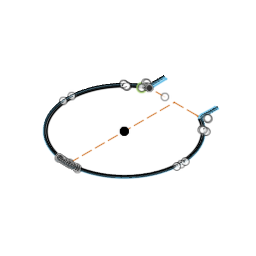
E-Baike Kunstoff abdeckung Schloss v12 (Autodesk Fusion 360 design; units mm, degrees)
Autodesk Fusion 360 part; units mm, degrees
note: some values were not read from the file. Set by a fixed rule: which sketch regions a step uses.
sketch "Skizze3" plane through (0, 0, 0) normal (0, 0, 1) x (1, 0, 0)
  line L0 (52.5263, 0.0019) -> (52.3815, 0.0019) construction
  line L1 (52.3815, 0.0019) -> (52.3815, -3.9178)
  line L2 (52.3815, 0.0019) -> (52.3815, 3.8983)
  arc A0 (37.2241, 37.4698) -> (37.51, 36.7698) centre (38.2241, 37.4698) ccw
  arc A1 (34.4473, 37.4285) -> (34.7597, 36.7024) centre (35.4473, 37.4285) ccw
  line L3 (-52.3815, 0.0019) -> (-52.3815, -3.9178)
  line L4 (-52.3815, 0.0019) -> (-52.3815, 3.8983)
  arc A2 (-34.7597, 36.7024) -> (-34.4473, 37.4285) centre (-35.4473, 37.4285) ccw
  arc A3 (-37.51, 36.7698) -> (-37.2241, 37.4698) centre (-38.2241, 37.4698) ccw
  line L5 (0, -50.55) -> (0, 46.165) construction
  line L6 (-25.0003, 48.4886) -> (-24.9973, 61.165)
  line L7 (25.0009, 48.4892) -> (25.0009, 61.165)
  line L8 (-24.9973, 61.165) -> (-24.3973, 61.1649)
  line L9 (25.0009, 61.165) -> (24.4009, 61.165)
  line L10 (23.8294, 48.6654) -> (24.4009, 61.165)
  line L11 (-23.8287, 48.6648) -> (-24.3973, 61.1649)
  line L12 (24.4009, 61.165) -> (22.5009, 61.165)
  line L13 (-24.3973, 61.1649) -> (-22.4973, 61.1644)
  arc A4 (-26.748, 42.8934) -> (-26.748, 42.8934) centre (0, 0) ccw
  arc A5 (-25.8336, 45.0137) -> (25.8341, 45.0134) centre (0, 0) ccw
  line L14 (-8.6883, 46.1611) -> (-20.5959, 46.164) construction
  line L15 (0, 46.165) -> (20.5936, 46.165) construction
  arc A6 (-25.8336, 45.0137) -> (-23.8287, 48.6648) centre (-27.8246, 48.483) ccw
  arc A7 (-26.9472, 45.0566) -> (-25.0003, 48.4886) centre (-29.0003, 48.4895) ccw
  arc A8 (25.0009, 48.4892) -> (26.9477, 45.0563) centre (29.0009, 48.4892) ccw
  arc A9 (23.8294, 48.6654) -> (25.8341, 45.0134) centre (27.8252, 48.4827) ccw
  line L16 (20.5936, 46.165) -> (22.0936, 46.165) construction
  line L17 (-20.5959, 46.164) -> (-22.0959, 46.164) construction
  line L18 (22.0936, 46.165) -> (22.0936, 45.4662) construction
  line L19 (-22.0959, 46.164) -> (-22.0959, 45.4651) construction
  line L20 (22.1899, 49.1795) -> (22.5009, 61.165)
  line L21 (-22.1908, 49.1767) -> (-22.4973, 61.1644)
  arc A10 (-25.198, 43.822) -> (25.1971, 43.8224) centre (0, 0) ccw
  arc A11 (52.3815, 3.5258) -> (26.9477, 45.0563) centre (0, 0) ccw
  arc A12 (-26.9472, 45.0566) -> (-52.3815, 3.5258) centre (0, 0) ccw
  arc A13 (-52.3815, -3.5258) -> (52.3815, -3.5258) centre (0, 0) ccw
  arc A14 (-25.198, 43.822) -> (-22.1908, 49.1767) centre (-28.1889, 49.0234) ccw
  arc A15 (22.1899, 49.1795) -> (25.1971, 43.8224) centre (28.1879, 49.0239) ccw
  line L22 (8.6033, -51.817) -> (8.6033, -51.7903) construction
  line L23 (-8.6033, -51.817) -> (-8.6033, -51.7903) construction
  point P0 (-25.0009, 46.165)
  point P1 (-25.0009, 46.165)
  point P2 (-25.7438, 46.1667)
  point P3 (-22.9574, 46.0854)
  dimension "d26" = 1
  dimension "d34" = 105
  dimension "d36" = 96.715
  dimension "d42" = 15
  dimension "d44" = 2.5
  dimension "d45" = 2.5
  dimension "d46" = 0.6
  dimension "d47" = 0.6
  dimension "d48" = 103.8
  dimension "d50" = 4
  dimension "d57" = 101.1
  dimension "d58" = 1.5
  dimension "d59" = 1.5
  dimension "d61" = 6
  dimension "d62" = 6
  constraint horizontal L0
  constraint perpendicular L0 L1
  constraint perpendicular L0 L2
  constraint equal A0 A1
  constraint coincident A4.centre A5.centre
  constraint perpendicular L5 L15
  constraint perpendicular L6 L14
  constraint perpendicular L7 L15
  constraint perpendicular L6 L8
  constraint perpendicular L7 L9
  constraint parallel L9 L12
  constraint parallel L8 L13
  constraint coincident A4 L14.end
  constraint tangent A5 A6
  constraint tangent L11 A6
  constraint tangent A7 A12
  constraint tangent L6 A7
  constraint equal A6 A7
  constraint tangent A8 A12
  constraint tangent L7 A8
  constraint equal A6 A8
  constraint tangent A5 A9
  constraint tangent L10 A9
  constraint equal A6 A9
  constraint coincident A7 P2
  constraint concentric A5 A10
  constraint parallel L15 L16
  constraint perpendicular L5 L17
  constraint perpendicular L16 L18
  constraint perpendicular L17 L19
  constraint coincident L19.end L21
  constraint coincident L19.end A10
  constraint coincident L18.end L20
  constraint coincident L18.end A10
  constraint coincident L1 A13.end
  constraint concentric A11 A12
  constraint coincident L2 A11.start
  constraint coincident L4 A12.end
  constraint coincident L3 A13.start
  constraint concentric A12 A13
  constraint tangent A10 A14
  constraint tangent L21 A14
  constraint midpoint A14 P3
  constraint tangent A10 A15
  constraint tangent L20 A15
  constraint coincident A13 L22.end
  constraint vertical L22
  constraint coincident A13 L23.end
  constraint vertical L23
  measures "d26" radius of A0
  measures "d34" diameter of A12
  measures "d36" distance of L5.start L5.end
  measures "d42" distance of P1 L6.end
  measures "d44" distance of L7.end L12.end
  measures "d45" distance of L6.end L13.end
  measures "d46" distance of L6.end L8.end
  measures "d47" distance of L7.end L9.end
  measures "d48" diameter of A5
  measures "d50" radius of A6
  measures "d57" diameter of A10
  measures "d58" distance of L15.end L16.end
  measures "d59" distance of L14.end L17.end
  measures "d61" radius of A14
  measures "d62" radius of A15
sketch "Skizze6" plane through (0, 0, 0) normal (0, 0, 1) x (1, 0, 0)
sketch "Skizze7" plane through (0, 0, 0) normal (0, 0, 1) x (1, 0, 0)
sketch "Skizze8" plane through (0, 0, 0) normal (0, 0, 1) x (1, 0, 0)
sketch "Skizze9" plane through (0, 0, 0) normal (0, 0, 1) x (1, 0, 0)
sketch "Skizze5" plane through (0, 0, 0) normal (0, 0, 1) x (1, 0, 0)
extrude "Extrusion4" add sketch "Skizze3" along normal blind 1.2 contours L1 L2 L3 L4 L6 L7 L8 L9 L10 L11 A5 A6 A7 A8 A9 A11 A12 A13
ref_plane "Arbeitsebene1" through (0.0001, 4.6324, 1) normal (0, 0, 1) x (1, 0, 0)
ref_plane "Arbeitsebene2" through (0.0001, 4.6324, 1) normal (0, 0, 1) x (1, 0, 0)
sketch "Skizze11" plane through (0, 0, 1) normal (0, 0, 1) x (1, 0, 0)
  line L0 (0, -54.5) -> (7, -54.5)
  line L1 (0, -54.5) -> (-7, -54.5)
  line L2 (-7, -54.5) -> (-8.4973, -51.8003)
  line L3 (7, -54.5) -> (8.3943, -51.8454)
  spline S0 degree 5 poles (8.3943, -51.8454) (8.3347, -51.8554) (8.2155, -51.8752) (8.0366, -51.9048) (7.7978, -51.9437) (7.4986, -51.9916) (7.1982, -52.0385) (6.8955, -52.0845) (6.5883, -52.1293) (6.2738, -52.1725) (5.9488, -52.2138) (5.6104, -52.2528) (5.2569, -52.2894) (4.8882, -52.3234) (4.507, -52.355) (4.1181, -52.3846) (3.7276, -52.4124) (3.3421, -52.4388) (2.9678, -52.4637) (2.6099, -52.4866) (2.2713, -52.5065) (1.9529, -52.5219) (1.6536, -52.5317) (1.3706, -52.5349) (1.0994, -52.5318) (0.8341, -52.5238) (0.568, -52.5138) (0.2945, -52.5047) (0.0084, -52.4989) (-0.2935, -52.4978) (-0.6109, -52.5002) (-0.9413, -52.5038) (-1.2805, -52.5058) (-1.6235, -52.5034) (-1.9654, -52.4948) (-2.302, -52.4801) (-2.6305, -52.4609) (-2.9491, -52.4396) (-3.2576, -52.4185) (-3.5566, -52.3992) (-3.8486, -52.382) (-4.1372, -52.3654) (-4.4259, -52.3474) (-4.7181, -52.3257) (-5.0153, -52.2991) (-5.3169, -52.2675) (-5.6202, -52.2324) (-5.9214, -52.1957) (-6.2166, -52.1596) (-6.5026, -52.1253) (-6.7782, -52.093) (-7.0437, -52.0615) (-7.3003, -52.0291) (-7.5498, -51.9938) (-7.7937, -51.9542) (-8.0328, -51.9092) (-8.2207, -51.8686) (-8.3597, -51.8355) (-8.4516, -51.8122) (-8.4973, -51.8003) knots 0 0 0 0 0 0 0.018182 0.036364 0.054545 0.072727 0.090909 0.109091 0.127273 0.145455 0.163636 0.181818 0.2 0.218182 0.236364 0.254545 0.272727 0.290909 0.309091 0.327273 0.345455 0.363636 0.381818 0.4 0.418182 0.436364 0.454545 0.472727 0.490909 0.509091 0.527273 0.545455 0.563636 0.581818 0.6 0.618182 0.636364 0.654545 0.672727 0.690909 0.709091 0.727273 0.745455 0.763636 0.781818 0.8 0.818182 0.836364 0.854545 0.872727 0.890909 0.909091 0.927273 0.945455 0.963636 0.981818 1 1 1 1 1 1
  point P0 (0, -52.5)
  point P1 (6.9022, -52.0831)
  point P2 (5.1341, -52.3002)
  point P3 (2.8542, -52.4708)
  point P4 (1.2567, -52.5328)
  point P5 (-1.7211, -52.5)
  point P6 (-3.4116, -52.4088)
  point P7 (-4.823, -52.3157)
  point P8 (-6.2964, -52.1501)
  point P9 (-7.5, -52)
extrude "Extrusion6" add sketch "Skizze11" along normal blind 1
